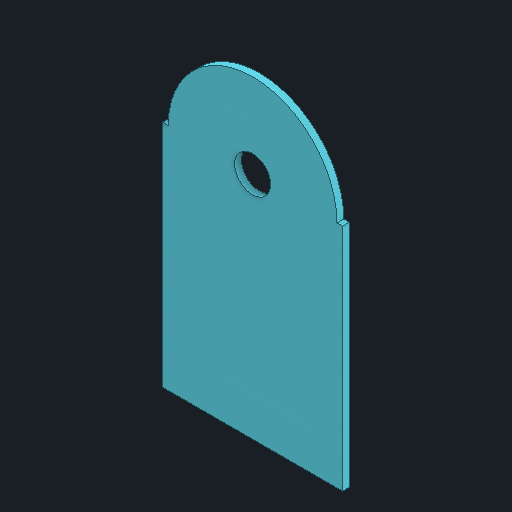
# Autodesk Inventor part: coxa_upper_steel
Saved by Autodesk Inventor 2026 (Build 300175000, 175)
## iProperties
Created: 2026-04-25
Part Number: coxa_upper_steel
Material: Сталь
Document SubType Name: Modeling
Designer: user
Mass: 282.6 g
Surface Area: 253.2 cm^2
Volume: 36 cm^3
Density: 7.85 g/cm^3
Appearance: Серо-синий
Author: user
Autodesk Inventor part; units mm, degrees
ref_plane "YZ Plane" through (0, 0, 0) normal (1, 0, 0) x (0, 1, 0)
ref_plane "XZ Plane" through (0, 0, 0) normal (0, 1, 0) x (-1, 0, 0)
ref_plane "XY Plane" through (0, 0, 0) normal (0, 0, 1) x (1, 0, 0)
sketch "Эскиз3" plane through (0, 0, 0) normal (0, 0, 1) x (1, 0, 0)
  line L0 (0, 0) -> (80, 0)
  line L1 (80, 0) -> (80, 102)
  line L2 (0, 102) -> (0, 0)
  circle A0 centre (40, 102) radius 8
  arc A1 (77.5, 102) -> (2.5, 102) centre (40, 102) ccw
  line L3 (80, 102) -> (77.5, 102)
  line L4 (2.5, 102) -> (0, 102)
  dimension "d8" = 102
  dimension "d9" = 80
  dimension "d10" = 16
  dimension "d11" = 75
  constraints: 10 end point, 3 parallel, 2 centre point, 2 horizontal alignment, 2 point on circle, 1 coincident, 1 collinear, 1 horizontal, 1 perpendicular
  measures "d8" distance of L2.start L0.start
  measures "d9" distance between parallel lines of L2 L1
  measures "d10" diameter of A0
  measures "d11" diameter of A1
extrude "Выдавливание3" add sketch "Эскиз3" along normal blind 3
equation "\"d9\" = width_coxa"
equation "\"d10\" = d_main_shaft"
equation "\"d6\" = thickness_steel"
equation "\"tolerance_plazma\" = 0.1"
equation "\"thickness_steel\" = 3"
equation "\"d_main_screw_holes\" = 6.1"
equation "\"d_main_shaft\" = 16"
equation "\"thickness_profile_tibea\" = 4"
equation "\"thickness_profile_femur\" = 3"
equation "\"width_shaft_shift\" = 35"
equation "\"width_flattened_surface\" = 12"
equation "\"width_coxa\" = 80"
